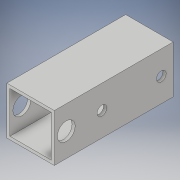
# Autodesk Inventor part: Front support bearing and stopper
Saved by Autodesk Inventor 2018 (Build 220112000, 112)
## iProperties
Created: 2019-03-20
Part Number: Front support bearing and stopper
Material: Generic
Document SubType Name: Modeling
Designer: S-4008082
Density: 1 g/cm^3
Appearance: Default
Author: S-4008082
Autodesk Inventor part; units mm, degrees
ref_plane "YZ Plane" through (0, 0, 0) normal (1, 0, 0) x (0, 1, 0)
ref_plane "XZ Plane" through (0, 0, 0) normal (0, 1, 0) x (-1, 0, 0)
ref_plane "XY Plane" through (0, 0, 0) normal (0, 0, 1) x (1, 0, 0)
sketch "Sketch1" plane through (0, 0, 0) normal (0, 0, 1) x (1, 0, 0)
  line L0 (12.7, -12.7) -> (-12.7, -12.7)
  line L1 (-12.7, -12.7) -> (-12.7, 12.7)
  line L2 (-12.7, 12.7) -> (12.7, 12.7)
  line L3 (12.7, 12.7) -> (12.7, -12.7)
  line L4 (12.7, -12.7) -> (-12.7, 12.7) construction
  line L5 (-12.7, -12.7) -> (12.7, 12.7) construction
  line L6 (11.049, -11.049) -> (-11.049, -11.049)
  line L7 (-11.049, -11.049) -> (-11.049, 11.049)
  line L8 (-11.049, 11.049) -> (11.049, 11.049)
  line L9 (11.049, 11.049) -> (11.049, -11.049)
  line L10 (11.049, -11.049) -> (-11.049, 11.049) construction
  line L11 (-11.049, -11.049) -> (11.049, 11.049) construction
  point P0 (0, 0)
  dimension "d0" = 25.4
  dimension "d1" = 25.4
  dimension "d2" = 1.651
  constraints: 24 end point, 4 midpoint, 4 parallel, 2 horizontal, 2 perpendicular, 1 point on line
  measures "d0" horizontal distance of L0.start L1.end
  measures "d1" distance of L2.end L0.start
  measures "d2" distance between parallel lines of L2 L8
extrude "Extrusion1" add sketch "Sketch1" along normal blind 63.5
sketch "Sketch2" plane through (12.7, -12.7, 0) normal (1, 0, 0) x (0, 0, -1)
  circle A0 centre (-57.15, 12.7) radius 4.7625
  line L0 (-63.5, 0) -> (-63.5, 25.4) projected
  circle A1 centre (-6.35, 12.7) radius 2.5797
  circle A2 centre (-38.1, 12.7) radius 2.5797
  line L1 (0, 25.4) -> (0, 0) projected
  line L2 (0, 0) -> (-63.5, 0) projected
  point P0 (0, 12.7)
  dimension "d5" = 9.525
  dimension "d6" = 6.35
  dimension "d7" = 5.1594
  dimension "d8" = 5.1594
  dimension "d9" = 19.05
  dimension "d10" = 6.35
  dimension "d11" = 12.7
  dimension "d12" = 12.7
  dimension "d13" = 12.7
  constraints: 3 centre point
  measures "d5" diameter of A0
  measures "d6" distance from line of L0 A0.centre
  measures "d7" diameter of A2
  measures "d8" diameter of A1
  measures "d9" distance of A2.centre A0.centre
  measures "d10" distance from line of L1 A1.centre
  measures "d11" distance from line of L2 A2.centre
  measures "d12" distance from line of L2 A0.centre
  measures "d13" distance from line of L2 A1.centre
extrude "Extrusion2" cut sketch "Sketch2" against normal blind 50.8
equation "\"d8\" = d7"
equation "\"d12\" = d11"
equation "\"d13\" = d11"
body "Solid1"
